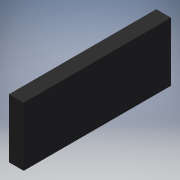
# Autodesk Inventor part: Rubber
Saved by Autodesk Inventor 2019 (Build 230136000, 136)
## iProperties
Created: 2020-02-25
Part Number: Rubber
Material: Generic
Document SubType Name: Modeling
Designer: USM
Density: 1 g/cm^3
Appearance: Rubber - Black
Author: USM
Autodesk Inventor part; units mm, degrees
ref_plane "YZ Plane" through (0, 0, 0) normal (1, 0, 0) x (0, 1, 0)
ref_plane "XZ Plane" through (0, 0, 0) normal (0, 1, 0) x (-1, 0, 0)
ref_plane "XY Plane" through (0, 0, 0) normal (0, 0, 1) x (1, 0, 0)
sketch "Sketch1" plane through (0, 0, 0) normal (1, 0, 0) x (0, 1, 0)
  line L0 (0, 0) -> (-20, 0)
  line L1 (-20, 0) -> (-20, -50)
  line L2 (-20, -50) -> (0, -50)
  line L3 (0, -50) -> (0, 0)
  dimension "d0" = 20
  dimension "d1" = 50
  constraints: 8 end point, 2 parallel, 1 horizontal, 1 perpendicular
  measures "d0" distance of L2.end L1.end
  measures "d1" distance of L1.end L0.end
extrude "Extrusion2" add sketch "Sketch1" along normal blind 5
body "Solid2"
